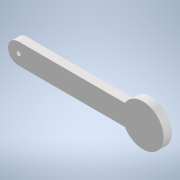
# Autodesk Inventor part: ShutterStop
Saved by Autodesk Inventor 2020.4 (Build 244396000, 396)
## iProperties
Created: 2021-10-26
Part Number: ShutterStop
Material: Generic
Document SubType Name: Modeling
Designer: TheLickerman
Density: 1 g/cm^3
Appearance: Default
Author: TheLickerman
Autodesk Inventor part; units mm, degrees
ref_plane "YZ Plane" through (0, 0, 0) normal (1, 0, 0) x (0, 1, 0)
ref_plane "XZ Plane" through (0, 0, 0) normal (0, 1, 0) x (-1, 0, 0)
ref_plane "XY Plane" through (0, 0, 0) normal (0, 0, 1) x (1, 0, 0)
sketch "Sketch1" plane through (0, 0, 0) normal (0, 0, 1) x (1, 0, 0)
  circle A0 centre (-14.45, 0) radius 0.6 projected
  line L0 (-14.45, 0) -> (23.65, 0) construction
  line L1 (-14.45, -3.175) -> (23.65, -3.175)
  line L2 (23.65, 3.175) -> (-14.45, 3.175)
  arc A1 (-14.45, 3.175) -> (-14.45, -3.175) centre (-14.45, 0) ccw
  arc A2 (23.65, -3.175) -> (23.65, 3.175) centre (23.65, 0) ccw
  line L3 (-14.45, 0) -> (23.65, 0) construction
  circle A3 centre (23.65, 0) radius 6.35
  point P0 (0, 0)
  point P1 (4.6, 0)
  point P2 (18.1507, -3.175)
  point P3 (18.1507, 3.175)
  dimension "d0" = 38.1
  dimension "d1" = 0
  dimension "d2" = 6.35
  dimension "d3" = 12.7
  constraints: 10 end point, 4 point on circle, 4 tangent, 3 centre point, 2 horizontal, 1 coincident, 1 collinear, 1 midpoint, 1 parallel
  measures "d0" distance of L0.start L0.end
  measures "d1" distance between parallel lines of L0 L3
  measures "d2" diameter of A2
  measures "d3" diameter of A3
extrude "Extrusion1" add sketch "Sketch1" along normal blind 2.54
body "Solid1"
